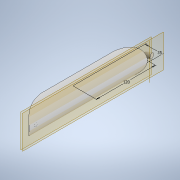
# Autodesk Inventor part: Deckel_Parachute_2
Saved by Autodesk Inventor 2020 (Build 240168000, 168)
## iProperties
Created: 2022-01-25
Part Number: Deckel_Parachute_2
Material: Generisch
Document SubType Name: Modeling
Designer: sp
Density: 1 g/cm^3
Appearance: Vorgabe
Author: sp
Autodesk Inventor part; units mm, degrees
ref_plane "XY Plane" through (0, 0, 0) normal (0, 0, 1) x (1, 0, 0)
sketch "Skizze1" plane through (0, 0, 0) normal (0, 0, 1) x (1, 0, 0)
  circle A0 centre (0, 0) radius 31
  circle A1 centre (0, 0) radius 30
  dimension "d0" = 62
  dimension "d1" = 60
  constraints: 2 centre point, 2 coincident
  measures "d0" diameter of A0
  measures "d1" diameter of A1
extrude "Extrusion1" add sketch "Skizze1" along normal mid plane 300
sketch "Skizze2" plane through (0, 0, 0) normal (0, 1, 0) x (-1, 0, 0)
  line L0 (-10, 169.5773) -> (-10, -169.8146) construction
  line L1 (-74.8376, 0) -> (82.6362, 0) construction
  line L2 (-10, 75) -> (-10, -75)
  line L3 (-31, -150) -> (-31, 150) projected
  line L4 (31, 150) -> (-31, 150) projected
  line L5 (-31, -150) -> (31, -150) projected
  spline S0 degree 2 poles (-10, 75) (-18.1599, 136.3675) (-72.8449, 128.3193) knots 0 0 0 1 1 1
  spline S1 degree 2 poles (-10, -75) (-17.9565, -136.1553) (-74.8376, -130) knots 0 0 0 1 1 1
  line L6 (-72.8449, 128.3193) -> (-74.8376, -130)
  line L7 (-31, 120) -> (-31, 150)
  line L8 (-31, 150) -> (31, 150)
  line L9 (31, 150) -> (31, -150)
  line L10 (31, -150) -> (31, 150) projected
  line L11 (31, -150) -> (-31, -150)
  line L12 (-31, -150) -> (-31, -120)
  point P0 (0, 0)
  dimension "d4" = 10
  dimension "d5" = 150
  dimension "d6" = 30
  dimension "d7" = 30
  constraints: 18 end point, 5 point on line, 3 perpendicular, 2 collinear, 1 horizontal, 1 symmetric about line, 1 vertical, 6 other
  measures "d4" distance from line of point (0, 0) L0
  measures "d5" distance of L2.start L2.end
  measures "d6" distance from line of L7.start L4
  measures "d7" distance from line of L12.end L5
extrude "Extrusion3" cut sketch "Skizze2" along normal mid plane 100 contours S0 L3 L4 L9 L5 S1 L2
ref_plane "Arbeitsebene1" through (26.5, 0, 0) normal (1, 0, 0) x (0, 1, 0)
sketch "Skizze3" plane through (26.5, 0, 0) normal (1, 0, 0) x (0, 1, 0)
  line L0 (0, 187.9338) -> (0, -197.3783) construction
  line L1 (-84.909, 0) -> (82.6972, 0) construction
  circle A0 centre (0, 106.5) radius 3.25
  point P0 (0, 0)
  dimension "d13" = 6.5
  dimension "d14" = 106.5
  constraints: 4 end point, 3 point on line, 1 centre point, 1 horizontal, 1 vertical
  measures "d13" diameter of A0
  measures "d14" distance of point (0, 0) A0.centre
extrude "Extrusion4" cut sketch "Skizze3" along normal blind 4
sketch "Skizze4" plane through (0, 0, 0) normal (0, 1, 0) x (-1, 0, 0)
  point P0 (0, 0)
  point P1 (-35, -120)
  dimension "d17" = 120
  dimension "d18" = 35
  measures "d17" vertical distance of point (-35, -120) point (0, 0)
  measures "d18" horizontal distance of point (0, 0) point (-35, -120)
ref_plane "Arbeitsebene2" through (30.5, 0, 0) normal (1, 0, 0) x (0, 1, 0)
sketch "Skizze5" plane through (30.5, 0, 0) normal (1, 0, 0) x (0, 1, 0)
  line L0 (-165.84, 0) -> (175.84, 0) construction
  line L1 (0, -526.424) -> (0, 61.2867) construction
  line L2 (-234.1759, -120) -> (244.1759, -120) projected
  circle A0 centre (0, -107) radius 5
  point P0 (0, 0)
  dimension "d24" = 10
  dimension "d25" = 107
  constraints: 4 end point, 3 point on line, 1 centre point, 1 horizontal, 1 vertical
  measures "d24" diameter of A0
  measures "d25" distance from line of L0 A0.centre
revolve "Umdrehung1" add sketch "Skizze5" angle 166 about axis through (30.5, 0, -120) along (0, -1, 0)
fillet "Rundung1" radius 3 3 edges at (29.7569, 3.8116, -103.781) (29.5804, -5, -107.0164) (29.757, 3.8109, -110.2652)
